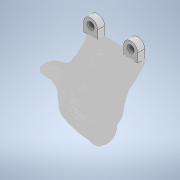
# Autodesk Inventor part: squirrel_head_small
Saved by Autodesk Inventor 2020 (Build 240168000, 168)
## iProperties
Created: 2019-05-04
Part Number: squirrel_head_small
Material: Generic
Document SubType Name: Modeling
Designer: mfans
Density: 1 g/cm^3
Appearance: Default
Author: mfans
Autodesk Inventor part; units mm, degrees
ref_plane "YZ Plane" through (0, 0, 0) normal (1, 0, 0) x (0, 1, 0)
ref_plane "XZ Plane" through (0, 0, 0) normal (0, 1, 0) x (-1, 0, 0)
ref_plane "XY Plane" through (0, 0, 0) normal (0, 0, 1) x (1, 0, 0)
sketch "Sketch1" plane through (-11.7708, 12.8725, 0) normal (0, 0, -1) x (-1, 0, 0)
  line L0 (3.043, 7.8767) -> (-29.111, 7.8767) projected
  line L1 (-27.2906, 7.8767) -> (-21.2906, 7.8767)
  line L2 (-21.2906, 7.8767) -> (-21.2906, 15.8767)
  line L3 (-21.2906, 15.8767) -> (-27.2906, 15.8767)
  line L4 (-27.2906, 15.8767) -> (-27.2906, 7.8767)
  line L5 (1.7094, 7.8767) -> (-4.2906, 7.8767)
  line L6 (-4.2906, 7.8767) -> (-4.2906, 15.8767)
  line L7 (-4.2906, 15.8767) -> (1.7094, 15.8767)
  line L8 (1.7094, 15.8767) -> (1.7094, 7.8767)
  point P0 (-11.7708, -12.8725)
  point P1 (-4.2906, 7.8767)
  dimension "d0" = 8
  dimension "d1" = 6
  dimension "d2" = 17
  constraints: 16 end point, 4 parallel, 3 point on line, 2 horizontal, 2 perpendicular, 1 collinear
  measures "d0" distance of L1.end L2.end
  measures "d1" distance of L2.end L3.end
  measures "d2" distance between parallel lines of L6 L2
extrude "Extrusion1" add sketch "Sketch1" against normal blind 4
fillet "Fillet1" radius 3 4 edges at (15.5198, 28.7492, 2) (9.5198, 28.7492, 2) (-7.4802, 28.7492, 2) (-13.4802, 28.7492, 2)
sketch "Sketch2" plane through (-11.7708, 12.8725, 4) normal (0, 0, 1) x (1, 0, 0)
  arc A0 (27.2906, 12.8767) -> (21.2906, 12.8767) centre (24.2906, 12.8767) ccw projected
  line L0 (21.2906, 12.8767) -> (21.2906, 7.8767) projected
  line L1 (21.2906, 7.8767) -> (27.2906, 7.8767) projected
  line L2 (27.2906, 7.8767) -> (27.2906, 12.8767) projected
  arc A1 (4.2906, 12.8767) -> (-1.7094, 12.8767) centre (1.2906, 12.8767) ccw projected
  line L3 (-1.7094, 12.8767) -> (-1.7094, 7.8767) projected
  line L4 (-1.7094, 7.8767) -> (4.2906, 7.8767) projected
  line L5 (4.2906, 7.8767) -> (4.2906, 12.8767) projected
  point P0 (11.7708, -12.8725)
  constraints: 2 coincident
hole "Hole1" at (12.5198, 25.7492, 4) at (-10.4802, 25.7492, 4) direction (0, 0, -1) diameter 4 end through all
thicken "Thicken1" operation add thickness 1 both sides no extend neighbours yes toward (0, 1, 0) faces at (-10.4802, 28.7492, 1.3333) (-12.1702, 28.2279, 1.3333) (-8.7902, 28.2279, 1.3333)
thicken "Thicken2" operation add thickness 1 both sides no extend neighbours yes toward (0, 1, 0) faces at (12.5198, 28.7492, 1.3333) (10.8298, 28.2279, 1.3333) (14.2098, 28.2279, 1.3333)
body "Solid1"
